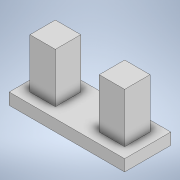
# Autodesk Inventor part: Keyboard_Prong
Saved by Autodesk Inventor 2021 (Build 250183000, 183)
## iProperties
Created: 2020-07-07
Part Number: Keyboard_Prong
Material: Generic
Document SubType Name: Modeling
Designer: ameli
Density: 1 g/cm^3
Appearance: Default
Author: ameli
Autodesk Inventor part; units mm, degrees
ref_plane "YZ Plane" through (0, 0, 0) normal (1, 0, 0) x (0, 1, 0)
ref_plane "XZ Plane" through (0, 0, 0) normal (0, 1, 0) x (-1, 0, 0)
ref_plane "XY Plane" through (0, 0, 0) normal (0, 0, 1) x (1, 0, 0)
sketch "Sketch1" plane through (0, 0, 0) normal (0, 1, 0) x (-1, 0, 0)
  line L0 (12.5, 5) -> (-12.5, 5)
  line L1 (-12.5, 5) -> (-12.5, -5)
  line L2 (-12.5, -5) -> (12.5, -5)
  line L3 (12.5, -5) -> (12.5, 5)
  point P0 (0, 0)
  dimension "d0" = 25
  dimension "d1" = 10
  dimension "d2" = 5
  dimension "d3" = 12.5
  constraints: 8 end point, 2 parallel, 1 horizontal, 1 perpendicular
  measures "d0" distance of L1.end L2.end
  measures "d1" distance of L2.end L0.start
  measures "d2" distance from line of point (0, 0) L0
  measures "d3" distance from line of L3 point (0, 0)
extrude "Extrusion1" add sketch "Sketch1" along normal blind 2.5
sketch "Sketch2" plane through (0, 2.5, 0) normal (0, 1, 0) x (1, 0, 0)
  line L0 (-10.25, -2.75) -> (-4.75, -2.75)
  line L1 (-4.75, -2.75) -> (-4.75, 2.75)
  line L2 (-4.75, 2.75) -> (-10.25, 2.75)
  line L3 (-10.25, 2.75) -> (-10.25, -2.75)
  line L4 (4.75, -2.75) -> (10.25, -2.75)
  line L5 (10.25, -2.75) -> (10.25, 2.75)
  line L6 (10.25, 2.75) -> (4.75, 2.75)
  line L7 (4.75, 2.75) -> (4.75, -2.75)
  line L8 (12.5, 5) -> (-12.5, 5) projected
  line L9 (12.5, -5) -> (12.5, 5) projected
  line L10 (-12.5, 5) -> (-12.5, -5) projected
  point P0 (0, 0)
  dimension "d6" = 2.25
  dimension "d7" = 2.25
  dimension "d8" = 2.25
  dimension "d9" = 2.25
  dimension "d10" = 5.5
  dimension "d11" = 5.5
  dimension "d12" = 5.5
  dimension "d13" = 5.5
  constraints: 16 end point, 4 parallel, 2 horizontal, 2 perpendicular
  measures "d6" distance between parallel lines of L8 L6
  measures "d7" distance between parallel lines of L9 L5
  measures "d8" distance between parallel lines of L10 L3
  measures "d9" distance between parallel lines of L8 L2
  measures "d10" distance of L2.end L0.start
  measures "d11" distance of L0.start L0.end
  measures "d12" distance of L6.end L4.start
  measures "d13" distance of L4.start L4.end
extrude "Extrusion2" add sketch "Sketch2" along normal blind 10.75
body "Solid1"
